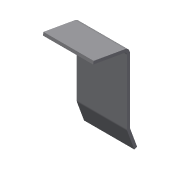
# Autodesk Inventor part: Claw - End piece
Saved by Autodesk Inventor 2015 (Build 190159000, 159)
## iProperties
Created: 2015-02-14
Part Number: Claw - End piece
Material: Generic
Document SubType Name: Sheet Metal
Designer: Tanner
Density: 1 g/cm^3
Sheet Metal Rule: Default
Appearance: Default
Author: Tanner
Autodesk Inventor part; units mm, degrees
ref_plane "YZ Plane" through (0, 0, 0) normal (1, 0, 0) x (0, 1, 0)
ref_plane "XZ Plane" through (0, 0, 0) normal (0, 1, 0) x (-1, 0, 0)
ref_plane "XY Plane" through (0, 0, 0) normal (0, 0, 1) x (1, 0, 0)
sketch "Sketch1" plane through (0, 0, 0) normal (0, 0, 1) x (1, 0, 0)
  line L0 (0, 0) -> (51.308, 0)
  line L1 (51.308, 0) -> (51.308, 126.746)
  line L2 (51.308, 126.746) -> (0, 126.746)
  line L3 (0, 126.746) -> (0, 0)
  dimension "d0" = 51.308
  dimension "d1" = 126.746
  measures "d0" distance of L2.end L1.end
  measures "d1" distance of L1.end L0.end
extrude "Plate1" add sketch "Sketch1" along normal blind 3.048
sketch "Sketch2" plane through (0, 0, 3.048) normal (0, 0, 1) x (1, 0, 0)
  line L0 (0, 91.186) -> (51.308, 91.186) construction
  line L1 (51.308, 0) -> (51.308, 126.746) construction
  line L2 (0, 126.746) -> (0, 0) construction
  line L3 (0, 78.74) -> (51.308, 78.74) construction
  line L4 (0, 21.59) -> (51.308, 21.59) construction
  line L5 (0, 126.746) -> (51.308, 126.746) construction
  dimension "d3" = 35.56
  dimension "d4" = 12.446
  dimension "d5" = 57.15
  dimension "d6" = 0
  constraints: 6 end point, 5 point on line, 1 horizontal, 1 parallel, 1 perpendicular
  measures "d3" distance between parallel lines of L5 L0
  measures "d4" distance between parallel lines of L3 L0
  measures "d5" distance between parallel lines of L3 L4
  measures "d6" distance from line of L2 L0.start
fold "Fold1" angle 80 bend radius 3.048 thickness 3.048 k factor 0.44 line from (0, 91.186, 3.048) to (51.308, 91.186, 3.048) line at bend centre moving side (0, 1, 0) folds toward (0, 0, 1)
sketch "Sketch4" plane through (0, 0, 0) normal (0, 0, -1) x (-1, 0, 0)
  line L0 (0, 21.59) -> (-51.308, 21.59) construction
  line L1 (-51.308, 0) -> (-51.308, 88.1218) construction
  line L2 (0, 0) -> (-51.308, 0) construction
  dimension "d21" = 21.59
  dimension "d22" = 51.308
  constraints: 2 end point, 1 horizontal, 1 point on line
  measures "d21" distance between parallel lines of L2 L0
  measures "d22" distance of L0.start L0.end
fold "Fold3" angle 20 bend radius 3.048 thickness 3.048 k factor 0.44 line from (0, 21.59, 0) to (51.308, 21.59, 0) line at bend centre moving side (0, -1, 0) folds toward (0, 0, -1)
equation "\"d7\" = BendReliefWidth"
equation "\"d8\" = BendReliefDepth"
equation "\"d9\" = MinimumRemnant"
equation "\"d10\" = BendRadius"
equation "\"d12\" = BendRadius"
equation "\"d23\" = BendReliefWidth"
equation "\"d24\" = BendReliefDepth"
equation "\"d25\" = MinimumRemnant"
equation "\"d26\" = BendRadius"
equation "\"d28\" = BendRadius"
equation "\"BendRadius\" = Thickness"
equation "\"BendReliefWidth\" = Thickness"
equation "\"BendReliefDepth\" = 0.5 * Thickness"
equation "\"CornerReliefSize\" = 4 * Thickness"
equation "\"MinimumRemnant\" = 2 * Thickness"
equation "\"TransitionRadius\" = BendRadius"
equation "\"JacobiRadiusSize\" = BendRadius"
equation "\"GapSize\" = Thickness"
equation "\"d2\" = BendRadius"
equation "\"Thickness\" = 3.048"
body "Solid1"
